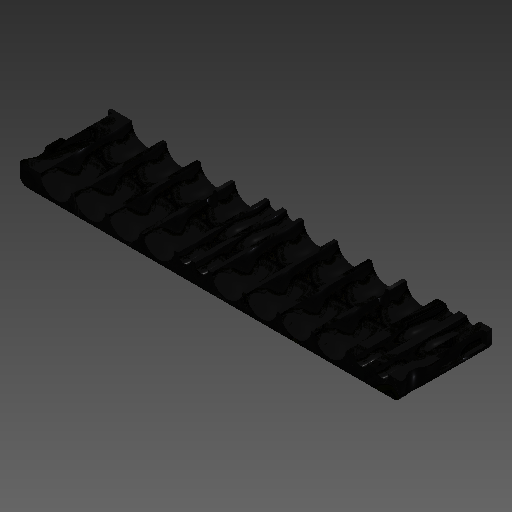
# Autodesk Inventor part: 3d_LM - Pinza 4
Saved by Autodesk Inventor 2018.3 (Build 223284000, 284)
## iProperties
Created: 2026-02-10
Part Number: 3d_LM - Pinza 4
Material: PA12 SLS 3D Print
Document SubType Name: Modeling
Designer: aca6
Density: 0.95 g/cm^3
Appearance: Black
Manufacturer-1: {"Name": "BERNARDO HENAREJOS ORENES (TECNOBRO)", "PartNumber": "3d_LM - Pinza 4", "Link": ""}
Manufacturer-2: {"Name": "MATERIALISE NV", "PartNumber": "3d_LM - Pinza 4", "Link": ""}
Manufacturer-3: {"Name": "", "PartNumber": "", "Link": ""}
Manufacturer-4: {"Name": "", "PartNumber": "", "Link": ""}
Manufacturer-5: {"Name": "", "PartNumber": "", "Link": ""}
Provider-1: {"Name": "", "PartNumber": "", "Link": ""}
Provider-2: {"Name": "", "PartNumber": "", "Link": ""}
Provider-3: {"Name": "", "PartNumber": "", "Link": ""}
Provider-4: {"Name": "", "PartNumber": "", "Link": ""}
Provider-5: {"Name": "", "PartNumber": "", "Link": ""}
Author: aca6
Comments: DIN-ISO-2768-mK
Autodesk Inventor part; units mm, degrees
ref_plane "YZ Plane" through (0, 0, 0) normal (1, 0, 0) x (0, 1, 0)
ref_plane "XZ Plane" through (0, 0, 0) normal (0, 1, 0) x (-1, 0, 0)
ref_plane "XY Plane" through (0, 0, 0) normal (0, 0, 1) x (1, 0, 0)
sketch "Sketch1" plane through (0, 0, 0) normal (0, 0, 1) x (1, 0, 0)
  line L0 (-25, 1.25) -> (-25, -0.25)
  line L1 (-24, -1.25) -> (24, -1.25)
  line L2 (25, -0.25) -> (25, 1.25)
  line L3 (25, 1.25) -> (-25, 1.25)
  line L4 (0, 0) -> (0, 5.9906) construction
  line L5 (0, 0) -> (2.2727, 0) construction
  arc A0 (-17.775, 1.25) -> (-13.725, 1.25) centre (-15.75, 1.25) ccw
  arc A1 (-13.275, 1.25) -> (-9.225, 1.25) centre (-11.25, 1.25) ccw
  arc A2 (-8.775, 1.25) -> (-4.725, 1.25) centre (-6.75, 1.25) ccw
  arc A3 (-4.255, 1.25) -> (-2.535, 1.25) centre (-3.395, 1.25) ccw
  arc A4 (-1.965, 1.25) -> (-0.245, 1.25) centre (-1.105, 1.25) ccw
  arc A5 (0.225, 1.25) -> (4.275, 1.25) centre (2.25, 1.25) ccw
  arc A6 (4.725, 1.25) -> (8.775, 1.25) centre (6.75, 1.25) ccw
  arc A7 (9.225, 1.25) -> (13.275, 1.25) centre (11.25, 1.25) ccw
  arc A8 (13.725, 1.25) -> (17.775, 1.25) centre (15.75, 1.25) ccw
  arc A9 (18.925, 1.25) -> (20.675, 1.25) centre (19.8, 1.25) ccw
  arc A10 (21.625, 1.25) -> (23.375, 1.25) centre (22.5, 1.25) ccw
  arc A11 (-25, -0.25) -> (-24, -1.25) centre (-24, -0.25) ccw
  arc A12 (24, -1.25) -> (25, -0.25) centre (24, -0.25) ccw
  arc A13 (-22.275, 1.25) -> (-18.225, 1.25) centre (-20.25, 1.25) ccw
  point P0 (-25, -1.25)
  point P1 (25, -1.25)
  dimension "d0" = 2.5
  dimension "d1" = 50
  dimension "d2" = 90
  dimension "d4" = 4.05
  dimension "d5" = 4.05
  dimension "d6" = 4.05
  dimension "d7" = 1.72
  dimension "d8" = 1.72
  dimension "d9" = 4.05
  dimension "d10" = 4.05
  dimension "d11" = 4.05
  dimension "d12" = 4.05
  dimension "d13" = 1.75
  dimension "d14" = 1.75
  dimension "d16" = 4.5
  dimension "d17" = 4.5
  dimension "d18" = 3.355
  dimension "d19" = 2.29
  dimension "d20" = 3.355
  dimension "d21" = 4.5
  dimension "d22" = 4.5
  dimension "d23" = 4.5
  dimension "d25" = 2.7
  dimension "d26" = 1
  dimension "d51" = 2.5
  dimension "d52" = 4.05
  dimension "d53" = 4.5
  dimension "d101" = 4.05
  constraints: 28 point on circle, 14 centre point, 10 end point, 4 point on line, 4 tangent, 3 vertical, 2 horizontal, 2 perpendicular, 1 equal radius, 1 parallel, 41 other
  measures "d0" distance of L0.start point (-25, -1.25)
  measures "d1" distance of point (-25, -1.25) point (25, -1.25)
  measures "d2" angle of L1 L0
  measures "d4" diameter of A0
  measures "d5" diameter of A1
  measures "d6" diameter of A2
  measures "d7" diameter of A3
  measures "d8" diameter of A4
  measures "d9" diameter of A5
  measures "d10" diameter of A6
  measures "d11" diameter of A7
  measures "d12" diameter of A8
  measures "d13" diameter of A9
  measures "d14" diameter of A10
  measures "d16" distance of A1.centre A0.centre
  measures "d17" distance of A2.centre A1.centre
  measures "d18" distance of A3.centre A2.centre
  measures "d19" distance of A4.centre A3.centre
  measures "d20" distance of A5.centre A4.centre
  measures "d21" distance of A6.centre A5.centre
  measures "d22" distance of A7.centre A6.centre
  measures "d23" distance of A8.centre A7.centre
  measures "d25" distance of A10.centre A9.centre
  measures "d26" radius of A11
  measures "d51" distance from line of L2 A10.centre
  measures "d52" diameter of A13
  measures "d53" distance of A13.centre A0.centre
  measures "d101" distance of A8.centre A9.centre
extrude "Extrusion1" add sketch "Sketch1" along normal blind 12 contours L3 A13 A0 A1 A2 A3 A4 A5 A6 A7 A8 A9 A10 L2 A12 L1 A11 L0
sketch "Sketch2" plane through (-24, -1.25, 0) normal (0, -1, 0) x (1, 0, 0)
  line L0 (49, 0) -> (49, 12) projected
  line L1 (-1, 0) -> (-1, 12) projected
  line L2 (0, 0) -> (48, 0) projected
  line L3 (-0.714, 0.4) -> (48.714, 0.4)
  line L4 (48.714, 1) -> (-0.714, 1)
  line L5 (48.714, 5) -> (-0.714, 5)
  line L6 (-0.714, 5) -> (-0.714, 5.6)
  line L7 (-0.714, 5.6) -> (48.714, 5.6)
  line L8 (48.714, 5.6) -> (48.714, 5)
  line L9 (-0.714, 1) -> (-0.714, 0.4)
  line L10 (48.714, 1) -> (48.714, 0.4)
  point P0 (24, 0)
  point P1 (37.5, 3)
  point P2 (15, 3)
  point P3 (48.714, 5.3)
  dimension "d29" = 11.5
  dimension "d30" = 22.5
  dimension "d32" = 3
  dimension "d33" = 0.6
  dimension "d34" = 0.6
  dimension "d35" = 0.4
  dimension "d36" = 4
  dimension "d48" = 0.286
  dimension "d49" = 0.6
  dimension "d50" = 0.286
  constraints: 16 end point, 4 point on line, 2 horizontal, 2 parallel, 2 vertical, 1 midpoint, 1 perpendicular
  measures "d29" distance from line of L0 point (37.5, 3)
  measures "d30" distance of point (15, 3) point (37.5, 3)
  measures "d32" distance from line of L2 point (15, 3)
  measures "d33" distance of L3.end L4.start
  measures "d34" distance of L7.end L5.start
  measures "d35" distance between parallel lines of L2 L3
  measures "d36" distance between parallel lines of L5 L4
  measures "d48" distance between parallel lines of L1 L6
  measures "d49" distance of L4.start L10.end
  measures "d50" distance between parallel lines of L0 L10
hole "Hole1" at (13.5, -1.25, 3) at (-9, -1.25, 3) direction (0, 1, 0) diameter 1.5 end through all
extrude "Extrusion3" cut sketch "Sketch2" against normal blind 0.3
sketch "Sketch3" plane through (0, 0, 0) normal (0, 0, -1) x (-1, 0, 0)
  line L0 (-23, 1.25) -> (-1.5933, 1.25)
  line L1 (-1.5933, 1.25) -> (-1.5933, 1.075)
  line L2 (-1.5933, 1.075) -> (-23, 1.075)
  line L3 (-23, 1.075) -> (-23, 1.25)
  line L4 (7.4905, 1.25) -> (21.4905, 1.25)
  line L5 (21.4905, 1.25) -> (21.4905, 1.075)
  line L6 (21.4905, 1.075) -> (7.4905, 1.075)
  line L7 (7.4905, 1.075) -> (7.4905, 1.25)
  line L8 (8.775, 1.25) -> (9.225, 1.25) projected
  line L9 (-25, -0.25) -> (-25, 1.25) projected
  line L10 (25, 1.25) -> (25, -0.25) projected
  point P0 (0, 0)
  point P1 (9, 1.25)
  dimension "d54" = 0.175
  dimension "d55" = 0.175
  dimension "d56" = 14
  dimension "d57" = 21.4067
  dimension "d58" = 2
  dimension "d59" = 3.5095
  constraints: 16 end point, 4 parallel, 2 horizontal, 2 perpendicular, 2 point on line, 1 midpoint
  measures "d54" distance of L0.end L1.end
  measures "d55" distance of L4.end L5.end
  measures "d56" distance of L4.start L4.end
  measures "d57" distance of L0.start L0.end
  measures "d58" distance between parallel lines of L9 L3
  measures "d59" distance between parallel lines of L10 L5
extrude "Extrusion4" cut sketch "Sketch3" against normal blind 25.3
ref_plane "Work Plane1" through (0, 0, 1.25) normal (0, 0, -1) x (-1, 0, 0)
sketch "Sketch5" plane through (-24, -1.25, 12) normal (0, -1, 0) x (1, 0, 0)
  circle A0 centre (-2.4, -2.0003) radius 2
  circle A1 centre (50.4, -2.0003) radius 2
  line L0 (-1, -12) -> (-1, 0) projected
  line L1 (-1, 0) -> (-1, -0.572)
  line L2 (49, -12) -> (49, 0) projected
  line L3 (49, 0) -> (49, -0.572)
  point P0 (24, -12)
  dimension "d71" = 4
  dimension "d72" = 4
  dimension "d73" = 0.572
  dimension "d74" = 0.572
  dimension "d75" = 1.4
  dimension "d76" = 1.4
  constraints: 4 end point, 2 point on line, 6 other
  measures "d73" distance of L0.end L1.end
  measures "d74" distance of L2.end L3.end
  measures "d75" horizontal distance of L3.end point (50.4, -2)
  measures "d76" distance from line of L0 point (-2.4, -2)
extrude "Extrusion6" cut sketch "Sketch5" against normal blind 4
ref_plane "Work Plane2" through (0, 0, 0.75) normal (0, 0, -1) x (-1, 0, 0)
sketch "Sketch6" plane through (0, 0, 0.75) normal (0, 0, -1) x (-1, 0, 0)
  line L0 (-25, 1.25) -> (-23.375, 1.25) projected
  line L1 (-25, 1.25) -> (-24.4, 1.25)
  line L2 (-24.4, 1.25) -> (-24.4, 0.5)
  line L3 (-24.4, 0.5) -> (-24.124, 0.5)
  line L4 (-24.124, 0.5) -> (-24.4667, -0.2996)
  line L5 (-24.124, 0.5) -> (-23.254, 0.5) construction
  line L6 (-24.4667, -0.2996) -> (-24.9987, -0.2996)
  line L7 (-24.4667, -0.2996) -> (-24.4, -0.2996) construction
  line L8 (-25, 1.25) -> (-25, -0.25) projected
  line L9 (-25, -0.25) -> (-25, 1.25) projected
  line L10 (-25, 1.25) -> (-25, -0.25)
  line L11 (-24.4, -0.2996) -> (-24.365, -0.2996)
  arc A0 (-24.714, -0.9501) -> (-24, -1.25) centre (-24, -0.25) ccw projected
  arc A1 (-25, -0.25) -> (-24.9987, -0.2996) centre (-24.0293, -0.25) ccw
  point P0 (0, 0)
  dimension "d80" = 0.6
  dimension "d81" = 0.75
  dimension "d82" = 0.276
  dimension "d83" = 113.2
  dimension "d84" = 0.87
  dimension "d86" = 0.532
  dimension "d87" = 180
  constraints: 18 end point, 4 horizontal, 4 point on line, 2 point on circle, 1 centre point, 1 collinear, 1 equal length, 1 perpendicular, 1 tangent
  measures "d80" distance of L0.start L1.end
  measures "d81" distance of L1.end L2.end
  measures "d82" distance of L2.end L3.end
  measures "d83" angle of L4 L5
  measures "d84" distance of L3.end L4.end
  measures "d86" distance of L4.end L6.end
  measures "d87" angle of L6 L7
extrude "Extrusion7" cut sketch "Sketch6" against normal blind 6.1
ref_plane "Work Plane3" through (0, 0, 0.45) normal (0, 0, -1) x (-1, 0, 0)
sketch "Sketch7" plane through (0, 0, 0.45) normal (0, 0, -1) x (-1, 0, 0)
  line L0 (-25, 1.25) -> (-24.25, 1.25)
  line L1 (-25, 1.25) -> (-24.4, 1.25)
  line L2 (-24.4, 1.25) -> (-24.4, 0.5)
  line L3 (-24.4, 0.5) -> (-24.124, 0.5)
  line L4 (-24.124, 0.5) -> (-24.4667, -0.2996)
  line L5 (-24.124, 0.5) -> (-23.254, 0.5) construction
  line L6 (-24.4667, -0.2996) -> (-24.9987, -0.2996)
  line L7 (-24.4667, -0.2996) -> (-24.4, -0.2996) construction
  line L8 (-25, 1.25) -> (-25, -0.25)
  line L9 (-25, -0.25) -> (-25, 1.25)
  line L10 (-25, 1.25) -> (-25, -0.25)
  line L11 (-24.4, -0.2996) -> (-24.365, -0.2996)
  arc A0 (-24.714, -0.9501) -> (-24, -1.25) centre (-24, -0.25) ccw
  arc A1 (-25, -0.25) -> (-24.9987, -0.2996) centre (-24.0293, -0.25) ccw
  line L12 (0, 0) -> (0, -6.4481) construction
  line L13 (25, 1.25) -> (24.25, 1.25)
  line L14 (24.4, 1.25) -> (24.4, 0.5)
  line L15 (24.4, 0.5) -> (24.124, 0.5)
  line L16 (24.124, 0.5) -> (23.254, 0.5) construction
  line L17 (24.4, -0.2996) -> (24.365, -0.2996)
  line L18 (24.4667, -0.2996) -> (24.4, -0.2996) construction
  line L19 (24.124, 0.5) -> (24.4667, -0.2996)
  line L20 (24.4667, -0.2996) -> (24.9987, -0.2996)
  arc A2 (24.9987, -0.2996) -> (25, -0.25) centre (24.0293, -0.25) ccw
  line L21 (25, 1.25) -> (25, -0.25)
  line L22 (25, 1.25) -> (25, -0.25)
  line L23 (25, -0.25) -> (25, 1.25)
  line L24 (25, 1.25) -> (24.4, 1.25)
  point P0 (24, -0.25)
  point P1 (24, -0.25)
  dimension "d92" = 0.6
  dimension "d93" = 0.75
  dimension "d94" = 0.276
  dimension "d95" = 113.2
  dimension "d96" = 0.87
  dimension "d97" = 0.532
  dimension "d98" = 180
  constraints: 50 end point, 14 symmetric about line, 8 point on line, 6 point on circle, 4 horizontal, 3 centre point, 2 vertical, 1 collinear, 1 equal length, 1 perpendicular, 1 tangent, 2 other
  measures "d92" distance of L0.start L2.start
  measures "d93" distance of L2.start L2.end
  measures "d94" distance of L2.end L3.end
  measures "d95" angle of L4 L5
  measures "d96" distance of L3.end L7.start
  measures "d97" distance of L7.start L6.end
  measures "d98" angle of L6 L7
extrude "Extrusion8" cut sketch "Sketch7" against normal blind 6.1 contours L21 A2 L20 L19 L15 L14 L13
body "Solid1"
